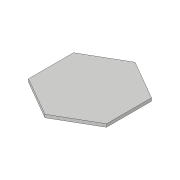
# Autodesk Inventor part: HEX_BASE
Saved by Autodesk Inventor 2017 (Build 210142000, 142)
## iProperties
Created: 2018-11-27
Part Number: HEX_BASE
Material: Generic
Document SubType Name: Modeling
Designer: jpb34
Density: 1 g/cm^3
Appearance: Default
Author: jpb34
Autodesk Inventor part; units mm, degrees
ref_plane "YZ Plane" through (0, 0, 0) normal (1, 0, 0) x (0, 1, 0)
ref_plane "XZ Plane" through (0, 0, 0) normal (0, 1, 0) x (-1, 0, 0)
ref_plane "XY Plane" through (0, 0, 0) normal (0, 0, 1) x (1, 0, 0)
sketch "Sketch1" plane through (0, 0, 0) normal (0, 1, 0) x (-1, 0, 0)
  line L0 (0, -190.5) -> (-164.9778, -95.25)
  line L1 (-164.9778, -95.25) -> (-164.9778, 95.25)
  line L2 (-164.9778, 95.25) -> (0, 190.5)
  line L3 (0, 190.5) -> (164.9778, 95.25)
  line L4 (164.9778, 95.25) -> (164.9778, -95.25)
  line L5 (164.9778, -95.25) -> (0, -190.5)
  point P0 (0, 0)
  point P1 (0, 0)
  dimension "d0" = 190.5
  constraints: 12 end point, 1 coincident, 13 other
  measures "d0" distance of L0.end L1.end
extrude "Extrusion1" add sketch "Sketch1" against normal blind 12.7
body "Solid1"
